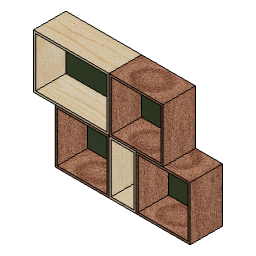
연습예제_5 (Autodesk Fusion 360 design; units mm, degrees)
Autodesk Fusion 360 part; units mm, degrees
sketch "Sketch1" plane through (0, 0, 0) normal (0, 1, 0) x (1, 0, 0)
  line L0 (0, 0) -> (250, 0)
  line L1 (250, 0) -> (250, -500)
  line L2 (250, -500) -> (0, -500)
  line L3 (0, -500) -> (0, 0)
  dimension "d1" = 250
  dimension "d2" = 500
  constraint horizontal L0
  constraint vertical L1
  constraint horizontal L2
  constraint vertical L3
  constraint coincident L0.start L3.end
  measures "d1" distance of L0.start L0.end
  measures "d2" distance of L0.start L2.end
sketch "Sketch2" plane through (0, 0, 0) normal (0, 1, 0) x (1, 0, 0)
  line L0 (250, 0) -> (750, 0)
  line L1 (750, 0) -> (750, -500)
  line L2 (750, -500) -> (250, -500)
  line L3 (250, -500) -> (250, 0)
  point P0 (250, 0)
  dimension "d3" = 500
  dimension "d4" = 500
  constraint horizontal L0
  constraint vertical L1
  constraint horizontal L2
  constraint vertical L3
  constraint coincident P0 L0.start
  measures "d3" distance of P0 L0.end
  measures "d4" distance of P0 L2.end
sketch "Sketch3" plane through (0, 0, 0) normal (0, 1, 0) x (1, 0, 0)
  line L0 (0, 0) -> (-500, 0)
  line L1 (-500, 0) -> (-500, -500)
  line L2 (-500, -500) -> (0, -500)
  line L3 (0, -500) -> (0, 0)
  dimension "d5" = 500
  dimension "d6" = 500
  constraint horizontal L0
  constraint vertical L1
  constraint horizontal L2
  constraint vertical L3
  constraint coincident L0.start L3.end
  measures "d5" distance of L0.start L0.end
  measures "d6" distance of L0.start L2.end
sketch "Sketch4" plane through (0, 0, 0) normal (0, 1, 0) x (1, 0, 0)
  line L0 (0, -500) -> (500, -500)
  line L1 (500, -500) -> (500, -1000)
  line L2 (500, -1000) -> (0, -1000)
  line L3 (0, -1000) -> (0, -500)
  point P0 (0, -500)
  dimension "d9" = 500
  dimension "d10" = 500
  constraint horizontal L0
  constraint vertical L1
  constraint horizontal L2
  constraint vertical L3
  constraint coincident P0 L0.start
  measures "d9" distance of P0 L0.end
  measures "d10" distance of P0 L2.end
sketch "Sketch5" plane through (0, 0, 0) normal (0, 1, 0) x (1, 0, 0)
  line L0 (0, -500) -> (-700, -500)
  line L1 (-700, -500) -> (-700, -1000)
  line L2 (-700, -1000) -> (0, -1000)
  line L3 (0, -1000) -> (0, -500)
  point P0 (0, -500)
  dimension "d11" = 700
  dimension "d12" = 500
  constraint horizontal L0
  constraint vertical L1
  constraint horizontal L2
  constraint vertical L3
  constraint coincident P0 L0.start
  measures "d11" distance of P0 L0.end
  measures "d12" distance of P0 L2.end
ref_plane "WorkPlane1" through (500, 300, 250) normal (0, 1, 0) x (1, 0, 0)
sketch "Sketch6" plane through (500, 300, 250) normal (0, 1, 0) x (1, 0, 0)
  line L0 (-250, -250) -> (250, -250)
  line L1 (250, -250) -> (250, 250)
  line L2 (250, 250) -> (-250, 250)
  line L3 (-250, 250) -> (-250, -250)
  line L4 (-500, -250) -> (-250, -250)
  line L5 (-250, -250) -> (-250, 250)
  line L6 (-250, 250) -> (-500, 250)
  line L7 (-500, 250) -> (-500, -250)
  line L8 (-1000, -250) -> (-500, -250)
  line L9 (-500, -250) -> (-500, 250)
  line L10 (-500, 250) -> (-1000, 250)
  line L11 (-1000, 250) -> (-1000, -250)
  line L12 (-500, -250) -> (0, -250)
  line L13 (0, -250) -> (0, -750)
  line L14 (0, -750) -> (-500, -750)
  line L15 (-500, -750) -> (-500, -250)
  line L16 (-500, -250) -> (-1200, -250)
  line L17 (-1200, -250) -> (-1200, -750)
  line L18 (-1200, -750) -> (-500, -750)
  line L19 (-500, -750) -> (-500, -250)
  point P0 (-250, -250)
  point P1 (250, 250)
  point P2 (-500, -250)
  point P3 (-1000, -250)
  point P4 (0, -750)
  point P5 (-1200, -750)
  constraint horizontal L0
  constraint vertical L1
  constraint horizontal L2
  constraint vertical L3
  constraint coincident P1 L1.end
  constraint coincident P0 L0.start
  constraint horizontal L4
  constraint vertical L5
  constraint horizontal L6
  constraint vertical L7
  constraint coincident P2 L4.start
  constraint horizontal L8
  constraint vertical L9
  constraint horizontal L10
  constraint vertical L11
  constraint coincident P3 L8.start
  constraint horizontal L12
  constraint vertical L13
  constraint horizontal L14
  constraint vertical L15
  constraint coincident P4 L13.end
  constraint coincident L4 P2
  constraint coincident L7 P2
  constraint horizontal L16
  constraint vertical L17
  constraint horizontal L18
  constraint vertical L19
  constraint coincident P5 L17.end
loft "Loft1" add profiles "Sketch6", "Sketch4" section 1 contours L0 L4 L12 L13 L14 L15 L19 section 2 makes body 1
loft "Loft2" add profiles "Sketch6", "Sketch5" section 1 contours L8 L15 L16 L17 L18 L19 section 2 separate body makes body 2
loft "Loft3" add profiles "Sketch6", "Sketch3" section 1 contours L7 L8 L9 L10 L11 L16 section 2 separate body makes body 3
loft "Loft4" add profiles "Sketch6", "Sketch1" section 1 contours L3 L4 L5 L6 L7 L9 L12 section 2 separate body makes body 4
loft "Loft5" add profiles "Sketch6", "Sketch2" section 1 contours L0 L1 L2 L3 L5 L12 section 2 separate body makes body 5
shell "Shell1" thickness 20 removed faces 5 at (250, 0, 833.3333) at (-400, 0, 833.3333) at (-333.3333, 0, 166.6667) at (83.3333, 0, 333.3333) at (500, 0, 166.6667) on bodies 1 2 3 4 5
